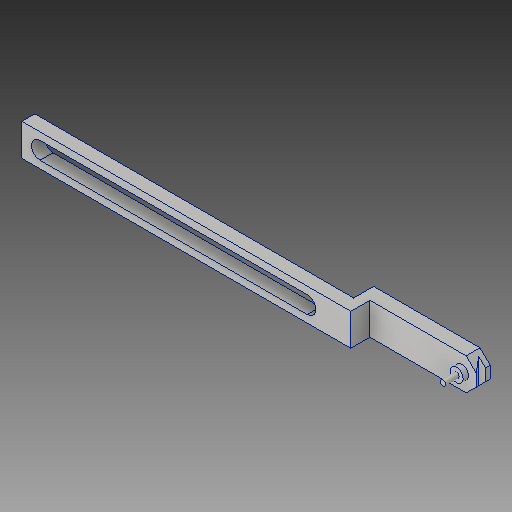
# Autodesk Inventor part: pinças
Saved by Autodesk Inventor 2018 (Build 220112000, 112)
## iProperties
Created: 2018-05-10
Part Number: pinças
Material: Alumínio 6061
Document SubType Name: Modeling
Designer: Georgines
Density: 2.7 g/cm^3
Appearance: Alumínio - Plano
Author: Georgines
Autodesk Inventor part; units mm, degrees
ref_plane "YZ Plane" through (0, 0, 0) normal (1, 0, 0) x (0, 1, 0)
ref_plane "XZ Plane" through (0, 0, 0) normal (0, 1, 0) x (-1, 0, 0)
ref_plane "XY Plane" through (0, 0, 0) normal (0, 0, 1) x (1, 0, 0)
sketch "Esboço1" plane through (0, 0, 0) normal (0, 1, 0) x (-1, 0, 0)
  line L0 (0, 5) -> (39.87, 5)
  line L1 (39.87, 5) -> (39.87, 12.15)
  line L2 (39.87, 12.15) -> (163.24, 12.15)
  line L3 (163.24, 12.15) -> (163.24, 7.27)
  line L4 (163.24, 7.27) -> (43.67, 7.27)
  line L5 (43.67, 7.27) -> (43.67, -0.21)
  line L6 (43.67, -0.21) -> (0, -0.21)
  line L7 (0, 5) -> (2.5, 5) construction
  line L8 (2.5, 5) -> (2.5, 1.56) construction
  line L9 (2.5, 1.56) -> (0, 1.56) construction
  line L10 (2.5, 1.56) -> (0, 5)
  line L11 (2.5, 1.56) -> (0, 1.56)
  line L12 (0, 1.56) -> (0, -0.21)
  point P0 (0, 0)
  dimension "d0" = 39.87
  dimension "d1" = 7.15
  dimension "d2" = 123.37
  dimension "d3" = 4.88
  dimension "d4" = 119.57
  dimension "d5" = 7.48
  dimension "d6" = 2.5
  dimension "d7" = 3.44
  dimension "d8" = 5.21
  constraints: 26 end point, 6 perpendicular, 1 collinear, 1 point on line, 1 vertical
  measures "d0" distance of L0.start L0.end
  measures "d1" distance of L0.end L1.end
  measures "d2" distance of L1.end L2.end
  measures "d3" distance of L2.end L3.end
  measures "d4" distance of L3.end L4.end
  measures "d5" distance of L4.end L5.end
  measures "d6" distance of L0.start L7.end
  measures "d7" distance of L7.end L8.end
  measures "d8" distance of L6.end L0.start
extrude "Extrusão1" add sketch "Esboço1" along normal mid plane 12
ref_plane "Plano de trabalho1" through (-163.24, 6, 12.15) normal (0, 0, 1) x (1, 0, 0)
ref_plane "Plano de trabalho2" through (-39.87, 6, 5) normal (0, 0, 1) x (1, 0, 0)
sketch "Esboço2" plane through (-163.24, 6, 12.15) normal (0, 0, 1) x (1, 0, 0)
  line L0 (123.37, 0) -> (123.37, -12) construction
  line L1 (123.37, -6) -> (110.26, -6) construction
  line L2 (0, 0) -> (0, -12) construction
  line L3 (0, -6) -> (3.56, -6) construction
  line L4 (110.26, -6) -> (0, -6) construction
  line L5 (3.56, -6) -> (110.26, -6) construction
  line L6 (6.785, -9.225) -> (107.035, -9.225)
  line L7 (107.035, -2.775) -> (6.785, -2.775)
  arc A0 (6.785, -2.775) -> (6.785, -9.225) centre (6.785, -6) ccw
  arc A1 (107.035, -9.225) -> (107.035, -2.775) centre (107.035, -6) ccw
  point P0 (163.24, -6)
  point P1 (55.13, -6)
  point P2 (56.91, -6)
  dimension "d13" = 13.11
  dimension "d14" = 3.56
  dimension "d16" = 6.45
  constraints: 16 end point, 6 point on circle, 4 midpoint, 4 tangent, 2 centre point, 2 collinear, 2 horizontal, 2 point on line, 1 parallel
  measures "d13" distance of L1.start L1.end
  measures "d14" distance of L3.start L3.end
  measures "d16" diameter of A1
extrude "Extrusão2" cut sketch "Esboço2" against normal blind 12
sketch "Esboço3" plane through (-39.87, 6, 5) normal (0, 0, 1) x (1, 0, 0)
  line L0 (-3.8, -12) -> (39.87, -12) construction
  line L1 (39.87, -12) -> (36.07, -12) construction
  line L2 (36.07, -12) -> (36.07, 0) construction
  line L3 (39.87, 0) -> (-3.8, 0) construction
  line L4 (39.87, -6) -> (39.87, -3.705) construction
  line L5 (39.87, 0) -> (39.87, -12) construction
  line L6 (39.87, -6) -> (39.87, -8.295) construction
  line L7 (39.87, -8.295) -> (36.07, -12)
  line L8 (39.87, -12) -> (36.07, -12)
  line L9 (39.87, -8.295) -> (39.87, -12)
  line L10 (36.07, 0) -> (39.87, -3.705)
  line L11 (39.87, 0) -> (39.87, -3.705)
  line L12 (39.87, 0) -> (36.07, 0)
  dimension "d19" = 3.8
  dimension "d20" = 2.295
  dimension "d21" = 2.295
  constraints: 20 end point, 4 point on line, 3 collinear, 2 perpendicular
  measures "d19" distance of L0.end L1.end
  measures "d20" distance of L4.start L4.end
  measures "d21" distance of L4.start L6.end
extrude "Extrusão3" cut sketch "Esboço3" against normal blind 12
sketch "Esboço4" plane through (-39.87, 6, 5) normal (0, 0, 1) x (1, 0, 0)
  line L0 (39.87, -6) -> (34.49, -6) construction
  circle A0 centre (34.49, -6) radius 2.5
  dimension "d24" = 5.38
  dimension "d25" = 5
  constraints: 2 end point, 1 centre point, 1 coincident, 1 horizontal
  measures "d24" distance of L0.start L0.end
  measures "d25" diameter of A0
extrude "Extrusão4" add sketch "Esboço4" along normal blind 2
sketch "Esboço5" plane through (-5.38, 0, 7) normal (0, 0, 1) x (1, 0, 0)
  circle A0 centre (0, 0) radius 1
  point P0 (5.38, 0)
  dimension "d28" = 2
  constraints: 1 centre point
  measures "d28" diameter of A0
extrude "Extrusão5" add sketch "Esboço5" along normal blind 5.13
